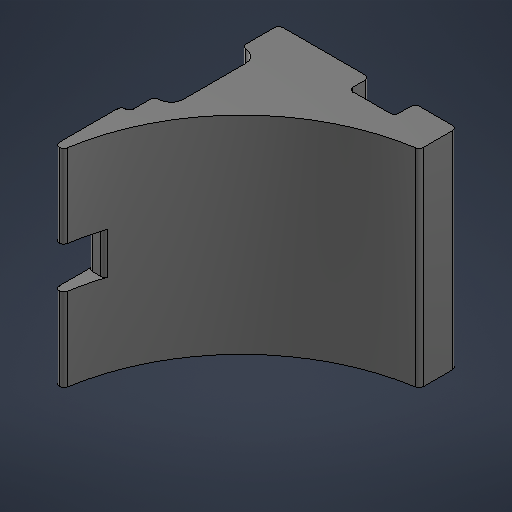
# Autodesk Inventor part: 3DPRINT,KICKER,RAMP
Saved by Autodesk Inventor 2026.1 (Build 301233020, 233B)
## iProperties
Created: 2026-02-08
Part Number: 3DPRINT,KICKER,RAMP
Material: ABS Plastic
Document SubType Name: Modeling
Designer: littl
Density: 0.189445 g/cm^3
Appearance: Smooth - Black
Mass: 250 g
Surface Area: 1050.21 cm^2
Volume: 1319.65 cm^3
Author: littl
Autodesk Inventor part; units mm, degrees
ref_plane "YZ Plane" through (0, 0, 0) normal (1, 0, 0) x (0, 1, 0)
ref_plane "XZ Plane" through (0, 0, 0) normal (0, 1, 0) x (-1, 0, 0)
ref_plane "XY Plane" through (0, 0, 0) normal (0, 0, 1) x (1, 0, 0)
sketch "Sketch1" plane through (0, 0, 0) normal (0, 1, 0) x (-1, 0, 0)
  line L0 (176.5377, -172.339) -> (176.5377, -7.239)
  line L1 (176.5377, -172.339) -> (-0.0024, -172.339)
  line L2 (20.2007, 67.3862) -> (178.9507, 67.3862) projected
  circle A0 centre (195.757, 2.286) radius 14.2875 projected
  circle A1 centre (195.757, 2.286) radius 25.4
  arc A2 (40.0127, -143.764) -> (176.5377, -7.239) centre (17.7877, 14.986) ccw
  line L3 (40.0127, -143.764) -> (40.0127, -172.339)
  line L4 (176.5377, -58.039) -> (182.8877, -58.039)
  line L5 (176.5377, -77.089) -> (163.8377, -77.089)
  line L6 (163.8377, -77.089) -> (163.8377, -143.764)
  line L7 (163.8377, -143.764) -> (176.5377, -143.764)
  line L8 (176.5377, -143.764) -> (176.5377, -77.089)
  circle A3 centre (17.7877, 14.986) radius 11.1125 projected
  line L9 (182.8877, -58.039) -> (182.8877, -7.239)
  line L10 (182.8877, 24.1845) -> (182.8877, 24.511)
  line L11 (176.5377, -7.239) -> (182.8877, -7.239)
  point P0 (0, 0)
  point P1 (23.4456, -172.339)
  dimension "d53" = 50.8
  dimension "d26" = 172.339
  dimension "d54" = 28.575
  dimension "d55" = 136.525
  dimension "d56" = 165.1
  dimension "d59" = 6.35
  dimension "d60" = 114.3
  dimension "d67" = 12.7
  dimension "d68" = 66.675
  dimension "d69" = 28.575
  dimension "d77" = 22.225
  constraints: 22 end point, 6 perpendicular, 4 point on line, 3 horizontal, 2 coincident, 2 parallel, 2 point on circle, 1 centre point, 3 other
  measures "d26" distance from line of point (0, 0) L1
  measures "d54" distance from line of L1 L3.start
  measures "d55" distance between parallel lines of L0 L3
  measures "d56" distance of L0.start L0.end
  measures "d59" distance of L4.start L4.end
  measures "d60" distance between parallel lines of L1 L4
  measures "d67" distance of L7.end L6.end
  measures "d68" distance of L6.end L5.end
  measures "d69" distance between parallel lines of L1 L7
  measures "d77" distance from line of A2.centre L3
extrude "Extrusion1" add sketch "Sketch1" along normal blind 158.75 contours L1 L3 A2 A1 L0 L5 L6 L7 | L0 A1 L9 L4 | A2 L0 A1 | L0 L11 L9 A1
ref_plane "Work Plane1" through (0, 79.375, 0) normal (0, -1, 0) x (1, 0, 0)
fillet "Fillet5" radius 3.175 9 edges at (-40.0127, 79.375, -143.764) (-176.5377, 79.375, -172.339) (-176.5377, 79.375, -58.039) (-182.8877, 79.375, -58.039) (-176.5377, 79.375, -77.089) (-176.5377, 79.375, -143.764) (-40.0127, 79.375, -172.339) (-182.8877, 79.375, -7.239) (-176.5377, 79.375, -7.239)
fillet "Fillet5" radius 9.525 2 edges at (-163.8377, 79.375, -77.089) (-163.8377, 79.375, -143.764)
sketch "Sketch9" plane through (-43.1877, 0, -172.339) normal (0, 0, -1) x (-1, 0, 0)
  line L0 (0, 158.75) -> (130.175, 158.75) projected
  line L1 (28.8925, 158.75) -> (63.8175, 158.75)
  line L2 (63.8175, 158.75) -> (63.8175, 142.875)
  line L3 (63.8175, 142.875) -> (28.8925, 142.875)
  line L4 (28.8925, 142.875) -> (28.8925, 158.75)
  line L5 (0, 0) -> (130.175, 0) projected
  line L6 (47.9425, 0) -> (82.8675, 0)
  line L7 (82.8675, 0) -> (82.8675, 15.875)
  line L8 (82.8675, 15.875) -> (47.9425, 15.875)
  line L9 (47.9425, 15.875) -> (47.9425, 0)
  point P0 (-43.1877, 0)
  point P1 (133.35, 158.75)
  point P2 (46.355, 142.875)
  point P3 (63.8175, 158.75)
  point P4 (65.405, 15.875)
  dimension "d71" = 34.925
  dimension "d72" = 15.875
  dimension "d73" = 86.995
  dimension "d76" = 67.945
  constraints: 16 end point, 6 parallel, 2 horizontal, 2 midpoint, 2 perpendicular, 2 point on line
  measures "d71" distance of L2.end L3.end
  measures "d72" distance of L1.end L2.end
  measures "d73" horizontal distance of point (133.35, 158.75) point (46.355, 142.875)
  measures "d76" horizontal distance of point (133.35, 158.75) point (65.405, 15.875)
extrude "Extrusion6" cut sketch "Sketch9" against normal blind 15.875
sketch "Sketch10" plane through (0, 79.375, 0) normal (0, -1, 0) x (1, 0, 0)
  line L0 (-157.4877, -7.239) -> (-182.8877, -7.239)
  line L1 (-182.8877, -7.239) -> (-182.8877, -32.639)
  line L2 (-182.8877, -32.639) -> (-157.4877, -32.639)
  line L3 (-157.4877, -32.639) -> (-157.4877, -7.239)
  line L4 (-157.4877, -7.239) -> (-182.8877, -32.639) construction
  line L5 (-182.8877, -7.239) -> (-157.4877, -32.639) construction
  line L6 (-107.0052, -172.339) -> (-173.3627, -172.339) projected
  line L7 (-182.8877, -54.864) -> (-182.8877, -10.414) projected
  point P0 (0, 0)
  point P1 (-170.1877, -19.939)
  dimension "d78" = 25.4
  dimension "d79" = 152.4
  constraints: 12 end point, 2 midpoint, 2 parallel, 2 perpendicular, 1 collinear, 1 horizontal
  measures "d78" distance of L0.start L0.end
  measures "d79" distance from line of L6 point (-170.188, -19.939)
extrude "Extrusion7" cut sketch "Sketch10" along normal mid plane 31.75
fillet "Fillet7" radius 3.175 10 edges at (-182.8877, 79.375, -32.639) (-170.8478, 79.375, -32.639) (-126.0552, 7.9375, -172.339) (-91.1302, 7.9375, -172.339) (-126.0552, 7.9375, -156.464) (-91.1302, 7.9375, -156.464) (-107.0052, 150.8125, -156.464) (-107.0052, 150.8125, -172.339) (-72.0802, 150.8125, -172.339) (-72.0802, 150.8125, -156.464)
body "Solid1"
